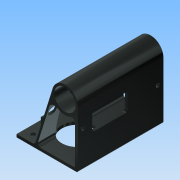
# Autodesk Inventor part: лЕВАЯ  КАРЕТКА  Y
Saved by Autodesk Inventor 2017 (Build 210142000, 142)
## iProperties
Part Number: лЕВАЯ  КАРЕТКА  Y
Material: Типовые
Document SubType Name: Modeling
Designer: Max
Mass: 16.1902 g
Surface Area: 179.517 cm^2
Volume: 16.1902 cm^3
Density: 1 g/cm^3
Appearance: Оружейный металл — полированный
Author: Max
Autodesk Inventor part; units mm, degrees
ref_plane "YZ Plane" through (0, 0, 0) normal (1, 0, 0) x (0, 1, 0)
ref_plane "XZ Plane" through (0, 0, 0) normal (0, 1, 0) x (-1, 0, 0)
ref_plane "XY Plane" through (0, 0, 0) normal (0, 0, 1) x (1, 0, 0)
sketch "Эскиз1" plane through (0, 0, 0) normal (0, 1, 0) x (-1, 0, 0)
  circle A0 centre (0, 0) radius 7.5
  line L0 (-9, 0) -> (-9, -40)
  line L1 (-9, -40) -> (34, -40)
  line L2 (34, -40) -> (34, -38)
  line L3 (17.0729, -38) -> (-6, -38)
  line L4 (-7, -37) -> (-7, -10.3562)
  line L5 (20.7636, -36.5921) -> (8.5966, 2.6644)
  line L6 (11.1548, -10.1499) -> (18.9833, -35.4079)
  line L7 (15.3422, -19.1) -> (29.7, -19.1)
  line L8 (29.7, -19.1) -> (29.7, -21.95)
  line L9 (29.7, -21.95) -> (16.2255, -21.95)
  line L10 (22, -37.883) -> (22, -40)
  arc A1 (-7, -37) -> (-6, -38) centre (-6, -37) ccw
  arc A2 (-4.1304, -8.5551) -> (5.1611, -7.9758) centre (0, 0) ccw
  arc A3 (8.5966, 2.6644) -> (-9, 0) centre (0, 0) ccw
  arc A4 (-4.1304, -8.5551) -> (-7, -10.3562) centre (-5, -10.3562) ccw
  arc A5 (11.1548, -10.1499) -> (5.1611, -7.9758) centre (7.3341, -11.334) ccw
  arc A6 (17.0729, -38) -> (18.9833, -35.4079) centre (17.0729, -36) ccw
  line L11 (22.674, -38) -> (22, -38)
  line L12 (22, -38) -> (34, -38)
  arc A7 (20.7636, -36.5921) -> (22.674, -38) centre (22.674, -36) ccw
  point P0 (-7, -6.4226)
  point P1 (21.2, -38)
  point P2 (8.9746, -3.1155)
  dimension "d0" = 15
  dimension "d3" = 2
  dimension "d4" = 2
  dimension "d5" = 43
  dimension "d6" = 12.8
  dimension "d7" = 1.35
  dimension "d8" = 2.85
  dimension "d9" = 38.7
  dimension "d10" = 31
  dimension "d11" = 20.9
  dimension "d12" = 1
  dimension "d13" = 9
  dimension "d14" = 40
  dimension "d15" = 49
  dimension "d16" = 2
  dimension "d17" = 2
  dimension "d18" = 4
  dimension "d19" = 2
  dimension "d20" = 2
  constraints: 26 end point, 17 point on circle, 12 tangent, 11 point on line, 8 centre point, 7 perpendicular, 2 coincident, 2 horizontal, 1 collinear, 1 parallel, 1 vertical
  measures "d0" diameter of A0
  measures "d3" distance between parallel lines of L0 L4
  measures "d4" distance between parallel lines of L1 L3
  measures "d5" distance between parallel lines of L2 L0
  measures "d6" distance from line of point (21.2, -38) L2
  measures "d7" distance between parallel lines of L6 L5
  measures "d8" distance between parallel lines of L9 L7
  measures "d9" distance between parallel lines of L0 L8
  measures "d10" distance between parallel lines of L0 L10
  measures "d11" distance between parallel lines of L7 L1
  measures "d12" radius of A1
  measures "d13" radius of A3
  measures "d14" distance from line of L1 point (0, 0)
  measures "d16" radial gap between concentric circles of A0 A2
  measures "d17" radius of A4
  measures "d18" radius of A5
  measures "d19" radius of A6
  measures "d20" radius of A7
extrude "Выдавливание1" add sketch "Эскиз1" against normal blind 60
sketch "Эскиз2" plane through (0, -60, 0) normal (0, -1, 0) x (1, 0, 0)
  arc A0 (-18.9833, -35.4079) -> (-17.0729, -38) centre (-17.0729, -36) ccw projected
  line L0 (-18.9833, -35.4079) -> (-11.1548, -10.1499) projected
  arc A1 (-5.1611, -7.9758) -> (-11.1548, -10.1499) centre (-7.3341, -11.334) ccw projected
  arc A2 (-5.1611, -7.9758) -> (4.1304, -8.5551) centre (0, 0) ccw projected
  arc A3 (7, -10.3562) -> (4.1304, -8.5551) centre (5, -10.3562) ccw projected
  line L1 (7, -10.3562) -> (7, -37) projected
  arc A4 (6, -38) -> (7, -37) centre (6, -37) ccw projected
  line L2 (6, -38) -> (-17.0729, -38) projected
  circle A5 centre (0, 0) radius 7.5 projected
  arc A6 (-22.674, -38) -> (-20.7636, -36.5921) centre (-22.674, -36) ccw projected
  line L3 (-22.674, -38) -> (-34, -38) projected
  line L4 (-34, -38) -> (-34, -40) projected
  line L5 (-34, -40) -> (9, -40) projected
  line L6 (9, -40) -> (9, 0) projected
  arc A7 (9, 0) -> (-8.5966, 2.6644) centre (0, 0) ccw projected
  line L7 (-8.5966, 2.6644) -> (-15.3422, -19.1) projected
  line L8 (-15.3422, -19.1) -> (-29.7, -19.1) projected
  line L9 (-29.7, -19.1) -> (-29.7, -21.95) projected
  line L10 (-29.7, -21.95) -> (-16.2255, -21.95) projected
  line L11 (-16.2255, -21.95) -> (-20.7636, -36.5921) projected
  line L12 (-15.3422, -19.1) -> (-29.7, -19.1) projected
  line L13 (-17, -19.1) -> (-17, -21.95)
  line L14 (-16.2255, -21.95) -> (-29.7, -21.95) projected
  dimension "d23" = 26
  constraints: 2 end point, 2 point on line, 1 vertical
  measures "d23" distance between parallel lines of L6 L13
extrude "Выдавливание2" cut sketch "Эскиз2" against normal blind 38 contours L10 L9 L8 L13
extrude "Выдавливание3" cut sketch "Эскиз1" against normal blind 17.5 contours L10 L11 L12 L2 L1 | L10 A7 L11
fillet "Сопряжение1" radius 2 1 edges at (-15.3422, -30, -19.1)
fillet "Сопряжение2" radius 2 1 edges at (-16.2255, -30, -21.95)
fillet "Сопряжение3" radius 1 1 edges at (9, -30, -40)
sketch "Эскиз3" plane through (0, 0, 0) normal (1, 0, 0) x (0, 1, 0)
  line L0 (-27, -8) -> (-48, -8)
  line L1 (-50, -10) -> (-50, -18.5)
  line L2 (-48, -20.5) -> (-27, -20.5)
  line L3 (-25, -18.5) -> (-25, -10)
  line L4 (-60, -7.5) -> (-60, 7.5) projected
  line L5 (0, 7.5) -> (0, -7.5) projected
  line L6 (-60, -40) -> (0, -40) projected
  line L7 (0, 9) -> (-60, 9) projected
  arc A0 (-25, -10) -> (-27, -8) centre (-27, -10) ccw
  arc A1 (-27, -20.5) -> (-25, -18.5) centre (-27, -18.5) ccw
  arc A2 (-50, -18.5) -> (-48, -20.5) centre (-48, -18.5) ccw
  arc A3 (-48, -8) -> (-50, -10) centre (-48, -10) ccw
  line L8 (-28, -20.5) -> (-31.5, -38)
  line L9 (-31.5, -38) -> (-45.5, -38)
  line L10 (0, -39) -> (-60, -39) projected
  line L11 (-45.5, -38) -> (-49, -20.5)
  line L12 (-60, -10.3562) -> (-60, -37) projected
  line L13 (-49, -20.5) -> (-49.0609, -20.1954)
  line L14 (0, -38) -> (-60, -38) projected
  line L15 (0, -38) -> (0, -37) projected
  line L16 (0, -38) -> (-60, -38) projected
  line L17 (-60, -37) -> (-60, -38) projected
  line L18 (0, -37) -> (-60, -37) projected
  line L19 (-38.5, -38) -> (-38.5, -31.8476) construction
  point P0 (0, 0)
  point P1 (-25, -8)
  point P2 (-50, -20.5)
  point P3 (-50, -8)
  point P4 (-25, -20.5)
  dimension "d31" = 25
  dimension "d32" = 12.5
  dimension "d33" = 10
  dimension "d34" = 25
  dimension "d35" = 19.5
  dimension "d36" = 17
  dimension "d39" = 2
  dimension "d40" = 11
  dimension "d41" = 21
  dimension "d42" = 14
  constraints: 18 end point, 10 point on line, 9 point on circle, 8 tangent, 4 centre point, 3 equal radius, 3 parallel, 2 collinear, 1 horizontal, 1 midpoint, 1 perpendicular, 1 vertical, 1 other
  measures "d31" distance between parallel lines of L1 L3
  measures "d32" distance between parallel lines of L2 L0
  measures "d33" distance between parallel lines of L4 L1
  measures "d34" distance between parallel lines of L5 L3
  measures "d35" distance between parallel lines of L6 L2
  measures "d36" distance between parallel lines of L0 L7
  measures "d39" radius of A0
  measures "d40" distance from line of L12 L11.end
  measures "d41" distance of L8.start L11.end
  measures "d42" distance of L8.end L9.end
extrude "Выдавливание4" cut sketch "Эскиз3" along normal mid plane 50 contours A0 L3 A1 L2 A2 L1 A3 L0
extrude "Выдавливание5" cut sketch "Эскиз3" against normal blind 50 contours A2 L2 L8 L18 L11 L13 | L8 L9 L11 L18
fillet "Сопряжение4" radius 0.2 2 edges at (-15.6814, -28, -20.5) (-15.6342, -49.0609, -20.1954)
sketch "Эскиз4" plane through (-22, -17.5, -40) normal (0, 0, -1) x (-1, 0, 0)
  circle A0 centre (-9.5, -21.25) radius 11
  line L0 (-25, -36.75) -> (6, -36.75) construction
  line L1 (6, -36.75) -> (6, -5.75) construction
  line L2 (6, -5.75) -> (-25, -5.75) construction
  line L3 (-25, -5.75) -> (-25, -36.75) construction
  line L4 (-25, -36.75) -> (6, -5.75) construction
  line L5 (6, -36.75) -> (-25, -5.75) construction
  circle A1 centre (6, -5.75) radius 1.5
  circle A2 centre (6, -36.75) radius 1.5
  circle A3 centre (-25, -36.75) radius 1.5
  circle A4 centre (-25, -5.75) radius 1.5
  line L6 (0.674, 0) -> (12, 0) projected
  line L7 (-31, 17.5) -> (-31, -42.5) projected
  line L8 (12, 0) -> (-31, 0)
  line L9 (-31, 0) -> (-31, -42.5)
  line L10 (-31, -42.5) -> (12, -42.5)
  line L11 (12, -42.5) -> (12, 0)
  line L12 (12, -21.25) -> (-15.7232, -21.25) construction
  line L13 (-3.0167, -42.5) -> (-10.8452, -42.5) projected
  line L14 (-9.5, -36.75) -> (-9.5, -8.0223) construction
  point P0 (-22, 17.5)
  point P1 (-9.5, -21.25)
  dimension "d46" = 22
  dimension "d47" = 31
  dimension "d48" = 31
  dimension "d49" = 3
  dimension "d50" = 3
  dimension "d51" = 3
  dimension "d52" = 3
  dimension "d55" = 43
  dimension "d56" = 21.5
  dimension "d57" = 21.5
  constraints: 24 end point, 6 midpoint, 5 centre point, 4 coincident, 4 parallel, 3 horizontal, 2 perpendicular, 2 point on line, 1 vertical
  measures "d46" diameter of A0
  measures "d47" distance of L2.end L1.end
  measures "d48" distance of L1.end L0.end
  measures "d49" diameter of A1
  measures "d50" diameter of A2
  measures "d51" diameter of A3
  measures "d52" diameter of A4
  measures "d55" distance between parallel lines of L7 L11
  measures "d56" distance between parallel lines of L11 L14
  measures "d57" distance between parallel lines of L7 L14
extrude "Выдавливание6" cut sketch "Эскиз4" against normal blind 15 contours A0 | A1 | A2 | A3 | A4
extrude "Выдавливание7" cut sketch "Эскиз4" against normal blind 25 contours A0
sketch "Эскиз5" plane through (0, 0, 0) normal (1, 0, 0) x (0, 1, 0)
  line L0 (-3.85, -15) -> (-56.15, -15) construction
  circle A0 centre (-56.15, -15) radius 1.5
  circle A1 centre (-3.85, -15) radius 1.5
  circle A2 centre (-3.85, -15) radius 3
  circle A3 centre (-56.15, -15) radius 3
  line L1 (0, 9) -> (-60, 9) projected
  line L2 (-60, -40) -> (0, -40) projected
  line L3 (0, -38) -> (-60, -38) projected
  line L4 (-30, 9) -> (-30, -12)
  line L5 (-60, -7.5) -> (-60, 7.5) projected
  line L6 (0, 7.5) -> (0, -7.5) projected
  circle A4 centre (-3.85, -15) radius 4 construction
  circle A5 centre (-56.15, -15) radius 4 construction
  point P0 (0, 0)
  dimension "d62" = 3
  dimension "d63" = 3
  dimension "d64" = 6
  dimension "d65" = 6
  dimension "d66" = 28
  dimension "d67" = 24
  dimension "d68" = 23
  dimension "d69" = 30
  dimension "d70" = 30
  dimension "d71" = 8
  dimension "d79" = 8
  dimension "d80" = 60.3
  dimension "d81" = 52.3
  constraints: 6 centre point, 6 coincident, 4 end point, 1 horizontal, 1 midpoint, 1 symmetric about line, 1 vertical
  measures "d62" diameter of A0
  measures "d63" diameter of A1
  measures "d64" diameter of A2
  measures "d65" diameter of A3
  measures "d67" distance from line of L1 L0.end
  measures "d68" distance from line of L0.end L3
  measures "d69" distance between parallel lines of L4 L5
  measures "d70" distance between parallel lines of L4 L6
  measures "d71" diameter of A4
  measures "d79" diameter of A5
  measures "d81" distance of L0.start L0.end
extrude "Выдавливание8" cut sketch "Эскиз5" along normal blind 25 contours A0 | A1
extrude "Выдавливание9" cut sketch "Эскиз5" against normal blind 25 contours A0 | A1 | A2 | A3
sketch "Эскиз6" plane through (-29.7, -22, -19.1) normal (0, 0, 1) x (1, 0, 0)
  line L0 (0, 22) -> (0, 0) projected
  line L1 (0, 18.55) -> (7, 18.55)
  line L2 (7, 18.55) -> (7, 14.55)
  line L3 (7, 14.55) -> (0, 14.55)
  line L4 (0, 14.55) -> (0, 18.55)
  line L5 (0, 22) -> (12.8838, 22) projected
  line L6 (0, 7.55) -> (7, 7.55)
  line L7 (7, 7.55) -> (7, 6)
  line L8 (7, 6) -> (0, 6)
  line L9 (0, 6) -> (0, 7.55)
  line L10 (0, 0) -> (12.7, 0) projected
  point P0 (29.7, 22)
  dimension "d86" = 7
  dimension "d87" = 3.45
  dimension "d88" = 4
  dimension "d89" = 7
  dimension "d90" = 6
  dimension "d91" = 1.55
  constraints: 16 end point, 4 parallel, 2 horizontal, 2 perpendicular, 2 point on line
  measures "d86" distance of L2.end L3.end
  measures "d87" distance between parallel lines of L5 L1
  measures "d88" distance between parallel lines of L3 L1
  measures "d89" distance between parallel lines of L3 L6
  measures "d90" distance between parallel lines of L8 L10
  measures "d91" distance between parallel lines of L8 L6
extrude "Выдавливание10" cut sketch "Эскиз6" against normal blind 5
sketch "Эскиз7" plane through (0, 0, 0) normal (1, 0, 0) x (0, 1, 0)
  line L0 (0, 0) -> (0, -39) projected
  line L1 (0, -4.7763) -> (-63.7813, -4.7763)
  line L2 (0, -7.5) -> (-60, -7.5) projected
  circle A0 centre (-14.8907, -4.7763) radius 1.5
  circle A1 centre (-48.8907, -4.7763) radius 1.5
  line L3 (-31.8907, -4.7763) -> (-31.8907, 4.2868)
  dimension "d94" = 3
  dimension "d95" = 3
  dimension "d96" = 34
  constraints: 4 end point, 3 point on line, 2 centre point, 1 midpoint, 1 parallel, 1 symmetric about line, 1 vertical
  measures "d94" diameter of A0
  measures "d95" diameter of A1
  measures "d96" distance of A1.centre A0.centre
extrude "Выдавливание11" cut sketch "Эскиз7" against normal blind 20
thread "Резьба1" size "M3x0.5" class "6H" standard "ANSI Metric M Profile" full length
thread "Резьба2" size "M3x0.5" class "6H" standard "ANSI Metric M Profile" full length
sketch "Эскиз9" plane through (-11.3676, -14.8907, -4.7763) normal (0, 1, 0) x (0, 0, 1)
  line L0 (1.5, 0) -> (1.5, 7.2618)
  line L1 (1.5, 7.2618) -> (1.1293, 7.2618)
  line L2 (1.1293, 7.2618) -> (1.1293, 0)
  line L3 (1.1293, 0) -> (1.5, 0)
  line L4 (0, -31.2324) -> (0, 28.9676) projected
  constraints: 8 end point
revolve "Вращение1" add sketch "Эскиз9" angle 360 about axis through (-11.3676, -14.8907, -4.7763) along (1, 0, 0) separate body
sketch "Эскиз8" plane through (-11.3676, -14.8907, -3.2763) normal (0, -1, 0) x (1, 0, 0)
  line L0 (-0.2918, -0.0255) -> (-0.2501, -0.0255) construction
  line L1 (0.0416, -0.3456) -> (-0.0001, -0.4257) construction
  line L2 (-0.5001, -0.4257) -> (-0.5418, -0.3456) construction
  line L3 (-0.2084, -0.0255) -> (-0.2501, 0.0546) construction
  line L4 (-0.2501, 0.0546) -> (-0.2918, -0.0255) construction
  line L5 (-0.5001, -0.4257) -> (-0.4584, -0.3456) construction
  line L6 (-0.2084, -0.0255) -> (-0.0418, -0.3456)
  line L7 (-0.5418, -0.3456) -> (-0.4584, -0.3456) construction
  arc A0 (-0.5418, -0.3456) -> (-0.5001, -0.3709) centre (-0.5001, -0.3239) ccw construction
  line L8 (0.0416, -0.3456) -> (-0.0418, -0.3456) construction
  line L9 (-0.5001, -0.4257) -> (-0.5001, -0.3456) construction
  line L10 (-0.0001, -0.4257) -> (-0.0001, -0.3456) construction
  line L11 (-0.2501, 0.0546) -> (-0.2501, -0.0002) construction
  line L12 (-0.5001, -0.3709) -> (-0.0001, -0.3709)
  arc A1 (-0.5001, -0.3709) -> (-0.4584, -0.3456) centre (-0.5001, -0.3239) ccw
  line L13 (-0.0418, -0.3456) -> (-0.0001, -0.4257) construction
  line L14 (-0.4584, -0.3456) -> (-0.2918, -0.0255)
  line L15 (-0.0001, -0.0002) -> (-0.0001, 0.0177)
  line L16 (-0.0001, 0.0177) -> (-0.0001, -0.0002)
  line L17 (-0.0001, -0.0002) -> (0.0334, -0.0002)
  arc A2 (-0.0418, -0.3456) -> (-0.0001, -0.3709) centre (-0.0001, -0.3239) ccw
  arc A3 (-0.0001, -0.3709) -> (0.0416, -0.3456) centre (-0.0001, -0.3239) ccw construction
  arc A4 (-0.2501, -0.0002) -> (-0.2918, -0.0255) centre (-0.2501, -0.0471) ccw
  arc A5 (-0.2084, -0.0255) -> (-0.2501, -0.0002) centre (-0.2501, -0.0471) ccw
  line L18 (-0.2501, -0.0002) -> (-0.2501, -0.0255) construction
  line L19 (-0.2501, -0.0255) -> (-0.2084, -0.0255) construction
  dimension "d103" = 55
  dimension "d104" = 0.08
  dimension "d105" = 0.08
  dimension "Эскиз8_ThreadOffset" = 0
  dimension "Эскиз8_MajorRadius" = 0.3707
  dimension "d108" = 0.5
  dimension "Эскиз8_MinorRadius" = 0
  constraints: 40 end point, 12 point on circle, 10 parallel, 8 tangent, 6 centre point, 6 collinear, 2 midpoint, 2 point on line, 1 horizontal, 1 perpendicular, 3 other
  measures "d103" angle of L6 L14
  measures "d104" distance of L3.end L0.end
  measures "d105" distance of L1.end L10.end
  measures "Эскиз8_ThreadOffset" distance between parallel lines of L15 L10
  measures "Эскиз8_MajorRadius" distance from line of L12 L15.start
  measures "d108" distance from line of L1.end L9
  measures "Эскиз8_MinorRadius" distance edge to line of A5 L17
coil "Пружина1" sketch "Эскиз8" operation cut axis through (-11.3676, -14.8907, -4.7763) along (1, 0, 0) pitch 0.5005 turns 16.506996 hand right bodies 2
sketch "Эскиз11" plane through (-11.3676, -48.8907, -4.7763) normal (0, 1, 0) x (0, 0, 1)
  line L0 (1.5, 0) -> (1.5, 7.2618)
  line L1 (1.5, 7.2618) -> (1.1293, 7.2618)
  line L2 (1.1293, 7.2618) -> (1.1293, 0)
  line L3 (1.1293, 0) -> (1.5, 0)
  line L4 (0, -31.2324) -> (0, 28.9676) projected
  constraints: 8 end point
revolve "Вращение2" add sketch "Эскиз11" angle 360 about axis through (-11.3676, -48.8907, -4.7763) along (1, 0, 0) separate body
sketch "Эскиз10" plane through (-11.3676, -48.8907, -3.2763) normal (0, -1, 0) x (1, 0, 0)
  line L0 (-0.2918, -0.0255) -> (-0.2501, -0.0255) construction
  line L1 (0.0416, -0.3456) -> (-0.0001, -0.4257) construction
  line L2 (-0.5001, -0.4257) -> (-0.5418, -0.3456) construction
  line L3 (-0.2084, -0.0255) -> (-0.2501, 0.0546) construction
  line L4 (-0.2501, 0.0546) -> (-0.2918, -0.0255) construction
  line L5 (-0.5001, -0.4257) -> (-0.4584, -0.3456) construction
  line L6 (-0.2084, -0.0255) -> (-0.0418, -0.3456)
  line L7 (-0.5418, -0.3456) -> (-0.4584, -0.3456) construction
  arc A0 (-0.5418, -0.3456) -> (-0.5001, -0.3709) centre (-0.5001, -0.3239) ccw construction
  line L8 (0.0416, -0.3456) -> (-0.0418, -0.3456) construction
  line L9 (-0.5001, -0.4257) -> (-0.5001, -0.3456) construction
  line L10 (-0.0001, -0.4257) -> (-0.0001, -0.3456) construction
  line L11 (-0.2501, 0.0546) -> (-0.2501, -0.0002) construction
  line L12 (-0.5001, -0.3709) -> (-0.0001, -0.3709)
  arc A1 (-0.5001, -0.3709) -> (-0.4584, -0.3456) centre (-0.5001, -0.3239) ccw
  line L13 (-0.0418, -0.3456) -> (-0.0001, -0.4257) construction
  line L14 (-0.4584, -0.3456) -> (-0.2918, -0.0255)
  line L15 (-0.0001, -0.0002) -> (-0.0001, 0.0177)
  line L16 (-0.0001, 0.0177) -> (-0.0001, -0.0002)
  line L17 (-0.0001, -0.0002) -> (0.0334, -0.0002)
  arc A2 (-0.0418, -0.3456) -> (-0.0001, -0.3709) centre (-0.0001, -0.3239) ccw
  arc A3 (-0.0001, -0.3709) -> (0.0416, -0.3456) centre (-0.0001, -0.3239) ccw construction
  arc A4 (-0.2501, -0.0002) -> (-0.2918, -0.0255) centre (-0.2501, -0.0471) ccw
  arc A5 (-0.2084, -0.0255) -> (-0.2501, -0.0002) centre (-0.2501, -0.0471) ccw
  line L18 (-0.2501, -0.0002) -> (-0.2501, -0.0255) construction
  line L19 (-0.2501, -0.0255) -> (-0.2084, -0.0255) construction
  dimension "d121" = 55
  dimension "d122" = 0.08
  dimension "d123" = 0.08
  dimension "Эскиз10_ThreadOffset" = 0
  dimension "Эскиз10_MajorRadius" = 0.3707
  dimension "d126" = 0.5
  dimension "Эскиз10_MinorRadius" = 0
  constraints: 40 end point, 12 point on circle, 10 parallel, 8 tangent, 6 centre point, 6 collinear, 2 midpoint, 2 point on line, 1 horizontal, 1 perpendicular, 3 other
  measures "d121" angle of L6 L14
  measures "d122" distance of L3.end L0.end
  measures "d123" distance of L1.end L10.end
  measures "Эскиз10_ThreadOffset" distance between parallel lines of L15 L10
  measures "Эскиз10_MajorRadius" distance from line of L12 L15.start
  measures "d126" distance from line of L1.end L9
  measures "Эскиз10_MinorRadius" distance edge to line of A5 L17
coil "Пружина2" sketch "Эскиз10" operation cut axis through (-11.3676, -48.8907, -4.7763) along (1, 0, 0) pitch 0.5005 turns 16.506996 hand right bodies 3
equation "\"d103\" = d110"
equation "\"d104\" = 0.160083 * Эскиз8_Pitch"
equation "\"d105\" = 0.160083 * Эскиз8_Pitch"
equation "\"d108\" = Эскиз8_Pitch"
equation "\"d121\" = d128"
equation "\"d122\" = 0.160083 * Эскиз10_Pitch"
equation "\"d123\" = 0.160083 * Эскиз10_Pitch"
equation "\"d126\" = Эскиз10_Pitch"
equation "\"d110\" = 55deg"
equation "\"Эскиз8_Pitch\" = 0.5"
equation "\"d128\" = 55deg"
equation "\"Эскиз10_Pitch\" = 0.5"
